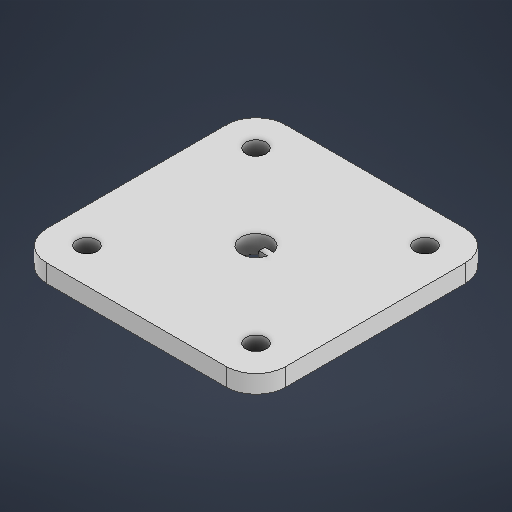
# Autodesk Inventor part: rod allingment
Saved by Autodesk Inventor 2025.2 (Build 292293000, 293)
## iProperties
Created: 2025-05-21
Part Number: rod allingment
Material: Generic
Document SubType Name: Modeling
Designer: klawy
Density: 1 g/cm^3
Appearance: Default
Author: klawy
Autodesk Inventor part; units mm, degrees
ref_plane "YZ Plane" through (0, 0, 0) normal (1, 0, 0) x (0, 1, 0)
ref_plane "XZ Plane" through (0, 0, 0) normal (0, 1, 0) x (-1, 0, 0)
ref_plane "XY Plane" through (0, 0, 0) normal (0, 0, 1) x (1, 0, 0)
sketch "Sketch1" plane through (0, 0, 0) normal (0, 1, 0) x (-1, 0, 0)
  circle A0 centre (0, 0) radius 14.5 construction
  circle A1 centre (0, 0) radius 2.5
  line L0 (-4, 0.5) -> (-1, 0.5)
  line L1 (-1, 0.5) -> (-1, -0.5)
  line L2 (-1, -0.5) -> (-4, -0.5)
  line L3 (-4, -0.5) -> (-4, 0.5)
  line L4 (-4, 0.5) -> (-1, -0.5) construction
  line L5 (-1, 0.5) -> (-4, -0.5) construction
  line L6 (20, 20) -> (-20, 20)
  line L7 (-20, 20) -> (-20, -20)
  line L8 (-20, -20) -> (20, -20)
  line L9 (20, -20) -> (20, 20)
  line L10 (20, 20) -> (-20, -20) construction
  line L11 (-20, 20) -> (20, -20) construction
  point P0 (-2.5, 0)
  point P1 (-2.4495, 0.5)
  point P2 (-2.4495, -0.5)
  dimension "d1" = 5
  dimension "d0" = 29
  dimension "d2" = 1
  dimension "d3" = 1
  dimension "d6" = 40
  dimension "d7" = 40
  constraints: 24 end point, 4 midpoint, 4 parallel, 2 coincident, 2 horizontal, 2 perpendicular, 1 centre point, 1 horizontal alignment, 3 other
  measures "d0" diameter of A0
  measures "d2" distance between parallel lines of L2 L0
  measures "d3" distance from line of point (0, 0) L1
  measures "d6" distance of L6.start L6.end
  measures "d7" distance of L8.end L6.start
extrude "Extrusion1" add sketch "Sketch1" along normal blind 3 contours L0 L1 L2 A1 | A1 L2 L3 L0 | L9 L8 L7 L6 picked at (-1.4981, -0.0559)
sketch "Sketch2" plane through (0, 3, 0) normal (0, 1, 0) x (1, 0, 0)
  arc A0 (2.4495, 0.5) -> (2.4495, -0.5) centre (0, 0) ccw projected
  line L0 (-20, 20) -> (-20, -20) projected
  circle A1 centre (0, 0) radius 20 construction
  line L1 (-20, -20) -> (0, 0) construction
  point P0 (-14.1421, -14.1421)
  point P1 (14.1421, -14.1421)
  point P2 (14.1421, 14.1421)
  point P3 (-14.1421, 14.1421)
  dimension "d8" = 40
  dimension "d11" = 360
  constraints: 2 end point, 1 coincident, 1 point on line, 8 other
hole "Hole1" at (-14.1421, 3, 14.1421) at (14.1421, 3, 14.1421) at (14.1421, 3, -14.1421) at (-14.1421, 3, -14.1421) direction (0, -1, 0) diameter 3.4 end through all clearance for "Socket Head Cap Screw ISO 4762" size "M3" standard "ISO"
fillet "Fillet1" radius 5 4 edges at (-20, 1.5, 20) (-20, 1.5, -20) (20, 1.5, -20) (20, 1.5, 20)
equation "\"d7\" = d6"
body "Solid1"
